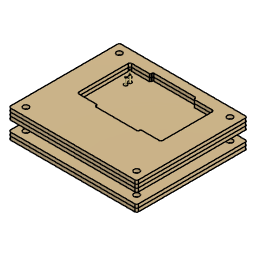
Hanshow Nebular 200-N - Fusion360 (Autodesk Fusion 360 design; units mm, degrees)
Autodesk Fusion 360 part; units mm, degrees
note: some values were not read from the file. Set by a fixed rule: which sketch regions a step uses.
sketch "Skizze1" plane through (0, 0, 0) normal (0, 0, 1) x (1, 0, 0)
  line L0 (-24.2511, -14.1981) -> (-24.2511, 14.4)
  line L1 (24.2501, 14.4) -> (24.2501, -14.1981)
  line L2 (12, -16.6981) -> (-12, -16.6981)
  line L3 (-12.5, -16.1981) -> (-12.5, -15.6981)
  line L4 (12.5, -15.6981) -> (12.5, -16.1981)
  line L5 (-12, 16.9) -> (12, 16.9)
  line L6 (12.5, 16.4) -> (12.5, 15.9)
  line L7 (-12.5, 15.9) -> (-12.5, 16.4)
  line L8 (25.25, 16.9) -> (-25.25, 16.9)
  line L9 (-25.25, 16.9) -> (-25.25, -35.4)
  line L10 (-25.25, -35.4) -> (25.25, -35.4)
  line L11 (25.25, -35.4) -> (25.25, 16.9)
  line L12 (-36, 22) -> (36, 22)
  line L13 (37, 21) -> (37, -41)
  line L14 (36, -42) -> (-36, -42)
  line L15 (-37, -41) -> (-37, 21)
  circle A0 centre (-32, 17) radius 1.6
  circle A1 centre (32, 17) radius 1.6
  circle A2 centre (-32, -37) radius 1.6
  circle A3 centre (32, -37) radius 1.6
  arc A4 (-36, 22) -> (-37, 21) centre (-36, 21) ccw
  arc A5 (37, 21) -> (36, 22) centre (36, 21) ccw
  arc A6 (-37, -41) -> (-36, -42) centre (-36, -41) ccw
  arc A7 (36, -42) -> (37, -41) centre (36, -41) ccw
  arc A8 (-23.2511, 15.4) -> (-24.2511, 14.4) centre (-23.2511, 14.4) ccw
  arc A9 (-24.2511, -14.1981) -> (-23.2511, -15.1981) centre (-23.2511, -14.1981) ccw
  arc A10 (24.2501, 14.4) -> (23.2501, 15.4) centre (23.2501, 14.4) ccw
  arc A11 (23.2501, -15.1981) -> (24.2501, -14.1981) centre (23.2501, -14.1981) ccw
  line L16 (-23.2511, 15.4) -> (-13, 15.4)
  line L17 (13, 15.4) -> (23.2501, 15.4)
  line L18 (23.2501, -15.1981) -> (13, -15.1981)
  line L19 (-13, -15.1981) -> (-23.2511, -15.1981)
  arc A12 (-13, 15.4) -> (-12.5, 15.9) centre (-13, 15.9) ccw
  arc A13 (12.5, 15.9) -> (13, 15.4) centre (13, 15.9) ccw
  arc A14 (12.5, 16.4) -> (12, 16.9) centre (12, 16.4) ccw
  arc A15 (-12, 16.9) -> (-12.5, 16.4) centre (-12, 16.4) ccw
  arc A16 (-12.5, -15.6981) -> (-13, -15.1981) centre (-13, -15.6981) ccw
  arc A17 (13, -15.1981) -> (12.5, -15.6981) centre (13, -15.6981) ccw
  arc A18 (-12.5, -16.1981) -> (-12, -16.6981) centre (-12, -16.1981) ccw
  arc A19 (12, -16.6981) -> (12.5, -16.1981) centre (12, -16.1981) ccw
  line L20 (0, 1.75) -> (0, 22.5)
  circle A20 centre (-20.95, 12) radius 1
  circle A21 centre (-18.41, 7.01) radius 1
  circle A22 centre (-18.41, 9.55) radius 1
  circle A23 centre (-20.95, 12) radius 0.45
  circle A24 centre (-18.41, 9.55) radius 0.45
  circle A25 centre (-18.41, 7.01) radius 0.45
  point P0 (-24.2511, -15.1981)
  point P1 (-24.2511, 15.4)
  point P2 (24.2501, 15.4)
  point P3 (-12.5, -16.6981)
  point P4 (-12.5, -15.1981)
  point P5 (12.5, -15.1981)
  point P6 (12.5, 16.9)
  point P7 (-12.5, 15.4)
  point P8 (-12.5, 16.9)
  dimension "d5" = 25
  dimension "d6" = 1.5
  dimension "d7" = 25
  dimension "d8" = 1.5
  dimension "d9" = 50.5
  dimension "d10" = 52.3
  dimension "d17" = 3.2
  dimension "d19" = 3.2
  dimension "d20" = 3.2
  dimension "d21" = 3.2
  dimension "d49" = 1
  dimension "d50" = 1
  dimension "d51" = 1
  dimension "d52" = 1
  dimension "d53" = 1
  dimension "d54" = 1
  dimension "d55" = 1
  dimension "d56" = 1
  dimension "d57" = 0.5
  dimension "d58" = 0.5
  dimension "d59" = 0.5
  dimension "d60" = 0.5
  dimension "d61" = 0.5
  dimension "d62" = 0.5
  dimension "d63" = 0.5
  dimension "d64" = 0.5
  constraint horizontal L18
  constraint perpendicular L0 L18
  constraint parallel L16 L18
  constraint parallel L0 L1
  constraint horizontal L2
  constraint perpendicular L2 L3
  constraint parallel L3 L4
  constraint parallel L6 L7
  constraint horizontal L8
  constraint perpendicular L8 L9
  constraint parallel L8 L10
  constraint parallel L9 L11
  constraint horizontal L12
  constraint vertical L13
  constraint horizontal L14
  constraint vertical L15
  constraint tangent L12 A4
  constraint tangent L15 A4
  constraint tangent L12 A5
  constraint tangent L13 A5
  constraint tangent L14 A6
  constraint tangent L15 A6
  constraint tangent L13 A7
  constraint tangent L14 A7
  constraint coincident P1 L0
  constraint coincident P1 L16
  constraint tangent L0 A8
  constraint tangent A8 L16
  constraint coincident P0 L18
  constraint coincident P0 L0
  constraint tangent A9 L18
  constraint tangent L0 A9
  constraint coincident P2 L16
  constraint coincident P2 L1
  constraint tangent A10 L16
  constraint tangent L1 A10
  constraint tangent A11 L18
  constraint tangent L1 A11
  constraint collinear L16 L17
  constraint collinear L18 L19
  constraint coincident P7 L7
  constraint coincident P7 L16
  constraint tangent L7 A12
  constraint tangent L16 A12
  constraint tangent L6 A13
  constraint tangent L17 A13
  constraint coincident P6 L5
  constraint coincident P6 L6
  constraint tangent L5 A14
  constraint tangent L6 A14
  constraint coincident P8 L5
  constraint coincident P8 L7
  constraint tangent L5 A15
  constraint tangent L7 A15
  constraint coincident P4 L3
  constraint coincident P4 L19
  constraint tangent L3 A16
  constraint tangent L19 A16
  constraint coincident P5 L4
  constraint coincident P5 L18
  constraint tangent L4 A17
  constraint tangent L18 A17
  constraint coincident P3 L2
  constraint coincident P3 L3
  constraint tangent L2 A18
  constraint tangent L3 A18
  constraint tangent L2 A19
  constraint tangent L4 A19
  measures "d5" distance of P4 P5
  measures "d6" distance of P3 P4
  measures "d7" distance of P6 P8
  measures "d8" distance of P7 P8
  measures "d9" distance of L9.end L10.end
  measures "d10" distance of L8.end L9.end
  measures "d17" diameter of A0
  measures "d19" diameter of A1
  measures "d20" diameter of A2
  measures "d21" diameter of A3
  measures "d49" radius of A4
  measures "d50" radius of A5
  measures "d51" radius of A6
  measures "d52" radius of A7
  measures "d53" radius of A8
  measures "d54" radius of A9
  measures "d55" radius of A10
  measures "d56" radius of A11
  measures "d57" radius of A12
  measures "d58" radius of A13
  measures "d59" radius of A14
  measures "d60" radius of A15
  measures "d61" radius of A16
  measures "d62" radius of A17
  measures "d63" radius of A18
  measures "d64" radius of A19
extrude "Extrusion25" add sketch "Skizze1" along normal blind 2 contours L0 L1 L2 L3 L4 L6 L7 L8 L9 L10 L11 A8 A9 A10 A11 L16 L17 L18 L19 A12 A13 A14 A15 A16 A17 A18 A19 | L0 L1 L2 L3 L4 L5 L6 L7 L8 A8 A9 A10 A11 L16 L17 L18 L19 A12 A13 A14 A15 A16 A17 A18 A19 | L12 L13 L14 L15 A4 A5 A6 A7 | A20 | A21 | A22 | A23 | A24 | A25 makes body 1
extrude "Extrusion26" add sketch "Skizze1" along normal blind 2 separate body contours L0 L1 L2 L3 L4 L6 L7 L8 L9 L10 L11 A8 A9 A10 A11 L16 L17 L18 L19 A12 A13 A14 A15 A16 A17 A18 A19 | L0 L1 L2 L3 L4 L5 L6 L7 L8 A8 A9 A10 A11 L16 L17 L18 L19 A12 A13 A14 A15 A16 A17 A18 A19 | L12 L13 L14 L15 A4 A5 A6 A7 | A20 | A21 | A22 makes body 2
move_body "Verschieben7" bodies 2 to x (1, 0, 0) y (0, 1, 0) z (0, 0, 1) at (0, 0, 2)
extrude "Extrusion27" add sketch "Skizze1" along normal blind 2 separate body contours L0 L1 L2 L3 L4 L6 L7 L8 L9 L10 L11 A8 A9 A10 A11 L16 L17 L18 L19 A12 A13 A14 A15 A16 A17 A18 A19 | L0 L1 L2 L3 L4 L5 L6 L7 L8 A8 A9 A10 A11 L16 L17 L18 L19 A12 A13 A14 A15 A16 A17 A18 A19 | L12 L13 L14 L15 A4 A5 A6 A7 makes body 3
move_body "Verschieben8" bodies 3 to x (1, 0, 0) y (0, 1, 0) z (0, 0, 1) at (0, 0, 10)
extrude "Extrusion28" add sketch "Skizze1" along normal blind 2 separate body contours L0 L1 L2 L3 L4 L6 L7 L8 L9 L10 L11 A8 A9 A10 A11 L16 L17 L18 L19 A12 A13 A14 A15 A16 A17 A18 A19 | L12 L13 L14 L15 A4 A5 A6 A7 makes body 4
move_body "Verschieben9" bodies 4 to x (1, 0, 0) y (0, 1, 0) z (0, 0, 1) at (0, 0, 12)
copy_body "Körper kopieren/einfügen2" bodies 4 makes body 5
move_body "Verschieben10" bodies 5 to x (1, 0, 0) y (0, 1, 0) z (0, 0, 1) at (0, 0, 2)
extrude "Extrusion31" add sketch "Skizze1" along normal blind 14 separate body contours A23 | A24 | A25 makes body 6 at (-20.7649, 12.4102, 9.3333) makes body 7 at (-18.2249, 9.9602, 9.3333) makes body 8 at (-18.2249, 7.4202, 9.3333)
move_body "Verschieben12" bodies 6 7 8 to x (1, 0, 0) y (0, 1, 0) z (0, 0, 1) at (0, 0, 2)
chamfer "Fase1" distance 0.3 angle 45 3 edges at (-18.8295, 6.8473, 16) (-21.3695, 11.8373, 16) (-18.8295, 9.3873, 16) on bodies 6 7 8
named bodies: "Layer 0", "Layer 1", "Layer 2", "Layer 3", "Layer 4", "Pin TX", "Pin RST", "Pin GND"
